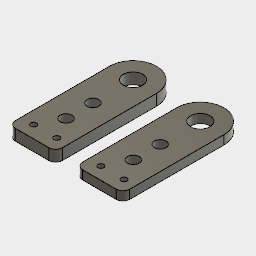
Idler_Bracket_v3 (Autodesk Fusion 360 design; units mm, degrees)
Autodesk Fusion 360 part; units mm, degrees
sketch "Sketch3" plane through (0, 0, 0) normal (0, 1, 0) x (1, 0, 0)
  line L0 (-5, 17) -> (16, 17)
  line L1 (16, 17) -> (16, -28)
  line L2 (16, -28) -> (-5, -28)
  line L3 (-5, -28) -> (-5, 17)
  circle A0 centre (5.5, 17) radius 10.5
  circle A1 centre (5.5, 17) radius 4.2768
  circle A2 centre (5.5112, -0.8825) radius 2.6
  circle A3 centre (5.5112, -12.8825) radius 2.6
  circle A4 centre (0.6669, -22.4594) radius 1.3
  circle A5 centre (10.9857, -22.4594) radius 1.3
  circle A6 centre (0.6669, -22.4594) radius 0.6
  circle A7 centre (10.9857, -22.4594) radius 0.6
  dimension "d1" = 1.2
  dimension "d2" = 1.2
  dimension "d3" = 2.6
  dimension "d4" = 2.6
  dimension "d5" = 5.2
  dimension "d6" = 5.2
  measures "d1" diameter of A6
  measures "d2" diameter of A7
  measures "d3" diameter of A5
  measures "d4" diameter of A4
  measures "d5" diameter of A3
  measures "d6" diameter of A2
extrude "Extrude1" add sketch "Sketch3" along normal blind 5 contours L0 A0 A1 | L0 A0 A1 | L1 L2 L3 A0 makes body 1
extrude "Extrude2" add sketch "Sketch3" along normal blind 2 contours A4 | A5 bodies 1
fillet "Fillet1" radius 3 2 edges at (16, 2.5, 28) (-5, 2.5, 28) on bodies 1
copy_body "CopyPasteBodies1" bodies 1 makes body 2
move_body "Move1" bodies 2 to x (1, 0, 0) y (0, 1, 0) z (0, 0, 1) at (30, 0, 0)
move_face "OffsetFaces1" offset -1 1 faces at (27.6467, 5, 3.09) on bodies 2
named bodies: "5mm", "4mm"
